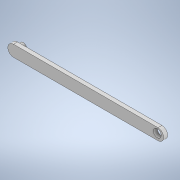
# Autodesk Inventor part: cranker rod part
Saved by Autodesk Inventor 2022 (Build 260153070, 153G)
## iProperties
Created: 2021-07-24
Part Number: cranker rod part
Material: Generic
Document SubType Name: Sheet Metal
Designer: DELL
Density: 1 g/cm^3
Sheet Metal Rule: Default
Appearance: Default
Author: DELL
Autodesk Inventor part; units mm, degrees
ref_plane "YZ Plane" through (0, 0, 0) normal (1, 0, 0) x (0, 1, 0)
ref_plane "XZ Plane" through (0, 0, 0) normal (0, 1, 0) x (-1, 0, 0)
ref_plane "XY Plane" through (0, 0, 0) normal (0, 0, 1) x (1, 0, 0)
sketch "Sketch1" plane through (0, 0, 0) normal (0, 0, 1) x (1, 0, 0)
  line L0 (-122.55, 8.89) -> (122.55, 8.89)
  line L1 (122.55, 8.89) -> (122.55, -8.89)
  line L2 (122.55, -8.89) -> (-122.55, -8.89)
  line L3 (-122.55, -8.89) -> (-122.55, 8.89)
  line L4 (-122.55, 8.89) -> (122.55, -8.89) construction
  line L5 (122.55, 8.89) -> (-122.55, -8.89) construction
  point P0 (0, 0)
  dimension "d0" = 245.1
  dimension "d1" = 17.78
  constraints: 12 end point, 2 midpoint, 2 parallel, 1 horizontal, 1 perpendicular
  measures "d0" distance of L1.end L2.end
  measures "d1" distance of L0.end L1.end
extrude "Extrusion1" add sketch "Sketch1" along normal blind 6.2
fillet "Fillet1" radius 8.89 1 edges at (122.55, 8.89, 3.1)
fillet "Fillet2" radius 8.89 1 edges at (122.55, -8.89, 3.1)
fillet "Fillet3" radius 8.89 1 edges at (-122.55, -8.89, 3.1)
fillet "Fillet4" radius 8.89 1 edges at (-122.55, 8.89, 3.1)
sketch "Sketch6" plane through (0, 0, 0) normal (0, 0, -1) x (-1, 0, 0)
  circle A0 centre (111.8854, 0) radius 5.5644
  point P0 (0, 0)
  constraints: 1 centre point
extrude "Extrusion4" add sketch "Sketch6" along normal blind 7.2
sketch "Sketch7" plane through (0, 0, 0) normal (0, 0, -1) x (-1, 0, 0)
  point P0 (0, 0)
  point P1 (-112.5539, 0.8007)
hole "Hole3" at (112.5539, 0.8007, 0) direction (0, 0, 1) diameter 12.4257 end through all
equation "\"BendRadius\" = Thickness"
equation "\"BendReliefWidth\" = Thickness"
equation "\"BendReliefDepth\" = 0.5 * Thickness"
equation "\"CornerReliefSize\" = 4 * Thickness"
equation "\"MinimumRemnant\" = 2 * Thickness"
equation "\"TransitionRadius\" = BendRadius"
equation "\"JacobiRadiusSize\" = BendRadius"
equation "\"GapSize\" = Thickness"
equation "\"Thickness\" = 3.048"
body "Solid1"
